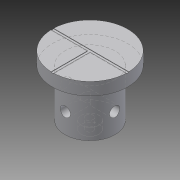
# Autodesk Inventor part: UNLHEP-14-01-P-008_ValveStopper
Saved by Autodesk Inventor 2013 (Build 170138000, 138)
## iProperties
Created: 2014-01-09
Part Number: UNLHEP-14-01-P-008_ValveStopper
Material: Allgemein
Document SubType Name: Modeling
Designer: Frank Meier
Density: 1 g/cm^3
Project: UNL Pixel Phase I
Author: Frank Meier
Revision Number: 00
Autodesk Inventor part; units mm, degrees
ref_plane "XY Plane" through (0, 0, 0) normal (0, 0, 1) x (1, 0, 0)
sketch "Skizze1" plane through (0, 0, 0) normal (0, 0, 1) x (1, 0, 0)
  circle A0 centre (0, 0) radius 9.975
  dimension "d0" = 19.95
  constraints: 1 centre point, 1 coincident
  measures "d0" diameter of A0
extrude "Extrusion1" add sketch "Skizze1" along normal blind 19
sketch "Skizze3" plane through (0, 0, 19) normal (0, 0, 1) x (1, 0, 0)
  circle A0 centre (0, 0) radius 15
  dimension "d8" = 30
  constraints: 1 centre point, 1 coincident
  measures "d8" diameter of A0
extrude "Extrusion3" add sketch "Skizze3" along normal blind 5
sketch "Skizze4" plane through (0, 0, 0) normal (0, 0, -1) x (-1, 0, 0)
  circle A0 centre (0, 0) radius 9.975 projected
  circle A1 centre (0, 0) radius 3.5
  dimension "d12" = 7
  constraints: 1 centre point, 1 coincident
  measures "d12" diameter of A1
extrude "Extrusion4" add sketch "Skizze4" along normal blind 3.1 contours A1
ref_plane "Arbeitsebene1" through (9.975, 0, 0) normal (1, 0, 0) x (0, 1, 0)
sketch "Skizze5" plane through (9.975, 0, 0) normal (1, 0, 0) x (0, 1, 0)
  circle A0 centre (0, 8) radius 2
  line L0 (-9.975, 0) -> (9.975, 0) projected
  point P0 (0, 0)
  dimension "d16" = 4
  dimension "d18" = 8
  constraints: 1 centre point
  measures "d16" diameter of A0
  measures "d18" distance from line of L0 A0.centre
extrude "Extrusion5" cut sketch "Skizze5" against normal blind 20
ref_plane "Arbeitsebene2" through (0, -9.975, 0) normal (0, 1, 0) x (-1, 0, 0)
sketch "Skizze6" plane through (0, -9.975, 0) normal (0, 1, 0) x (-1, 0, 0)
  circle A0 centre (0, 8) radius 2
  point P0 (0, 0)
  dimension "d21" = 4
  dimension "d23" = 8
  constraints: 1 centre point
  measures "d21" diameter of A0
  measures "d23" distance of point (0, 0) A0.centre
extrude "Extrusion6" cut sketch "Skizze6" along normal blind 10
hole "Bohrung1" at (-0.2115, -0.0513, -3.1) direction (0, 0, 1) diameter 3 depth 4 tip angle 118
thread "Gewinde1" size "M3x0.5" class "6H" standard "ISO Metric profile" full length
ref_plane "Arbeitsebene3" through (15, 0, 19) normal (1, 0, 0) x (0, 1, 0)
sketch "Skizze7" plane through (15, 0, 19) normal (1, 0, 0) x (0, 1, 0)
  line L0 (-0.5, 5) -> (0.5, 5)
  line L1 (0.5, 5) -> (0.5, 4.8)
  line L2 (0.5, 4.8) -> (-0.5, 4.8)
  line L3 (-0.5, 4.8) -> (-0.5, 5)
  line L4 (15, 5) -> (-15, 5) projected
  point P0 (0, -19)
  dimension "d37" = 0.2
  dimension "d39" = 1
  dimension "d40" = 0.5
  dimension "d41" = 0
  constraints: 8 end point, 2 parallel, 1 horizontal, 1 perpendicular
  measures "d37" distance of L0.end L1.end
  measures "d39" distance of L1.end L2.end
  measures "d40" horizontal distance of point (0, -19) L2.end
  measures "d41" distance between parallel lines of L4 L0
extrude "Extrusion7" cut sketch "Skizze7" against normal blind 30
ref_plane "Arbeitsebene4" through (0, -15, 19) normal (0, 1, 0) x (-1, 0, 0)
sketch "Skizze8" plane through (0, -15, 19) normal (0, 1, 0) x (-1, 0, 0)
  line L0 (-0.5, 5) -> (0.5, 5)
  line L1 (0.5, 5) -> (0.5, 4.8)
  line L2 (0.5, 4.8) -> (-0.5, 4.8)
  line L3 (-0.5, 4.8) -> (-0.5, 5)
  line L4 (15, 5) -> (-15, 5)
  point P0 (0, -19)
  point P1 (0, -19)
  dimension "d44" = 0.2
  dimension "d45" = 1
  dimension "d46" = 0.5
  dimension "d47" = 0
  constraints: 10 end point, 2 parallel, 1 horizontal, 1 perpendicular
  measures "d44" distance of L0.end L1.end
  measures "d45" distance of L1.end L2.end
  measures "d46" horizontal distance of point (0, -19) L2.end
  measures "d47" distance between parallel lines of L4 L0
extrude "Extrusion8" cut sketch "Skizze8" along normal blind 15
